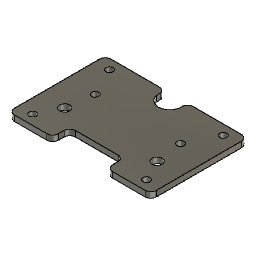
JRCNC0007 v3 (Autodesk Fusion 360 design; units mm, degrees)
Autodesk Fusion 360 part; units mm, degrees
sketch "Sketch1" plane through (0, 0, 0) normal (0, 0, 1) x (1, 0, 0)
  line L0 (-7.8581, 65) -> (-7.8581, 62)
  circle A0 centre (-40, 7) radius 2.5
  line L1 (-32.5, 22) -> (32.5, 22) construction
  line L2 (-40, 61) -> (-40, 7) construction
  arc A1 (19, 8) -> (15, 12) centre (15, 8) ccw
  line L3 (40, 7) -> (40, 61) construction
  arc A2 (-7.8581, 65) -> (-11.7311, 68) centre (-11.7311, 64) ccw
  arc A3 (-50, 4) -> (-46, 0) centre (-46, 4) ccw
  arc A4 (50, 64) -> (46, 68) centre (46, 64) ccw
  line L4 (19, 4) -> (19, 8)
  line L5 (7.8581, 65) -> (7.8581, 62)
  line L6 (-11.7311, 68) -> (-46, 68)
  circle A5 centre (32.5, 22) radius 3.6
  line L7 (-40, 7) -> (40, 7) construction
  line L8 (-30, 41) -> (30, 41) construction
  circle A6 centre (40, 61) radius 2.5
  circle A7 centre (40, 7) radius 2.5
  arc A8 (19, 4) -> (23, 0) centre (23, 4) ccw
  arc A9 (-46, 68) -> (-50, 64) centre (-46, 64) ccw
  line L9 (0, 0) -> (0, 50.832) construction
  arc A10 (11.7311, 68) -> (7.8581, 65) centre (11.7311, 64) ccw
  arc A11 (-15, 12) -> (-19, 8) centre (-15, 8) ccw
  line L10 (-50, 64) -> (-50, 4)
  arc A12 (-7.8581, 62) -> (7.8581, 62) centre (0, 63.5) ccw
  line L11 (15, 12) -> (-15, 12)
  circle A13 centre (-32.5, 22) radius 3.6
  arc A14 (-23, 0) -> (-19, 4) centre (-23, 4) ccw
  line L12 (23, 0) -> (46, 0)
  line L13 (46, 68) -> (11.7311, 68)
  line L14 (-50, 34) -> (50, 34) construction
  circle A15 centre (-30, 41) radius 2.5
  circle A16 centre (-40, 61) radius 2.5
  line L15 (40, 61) -> (-40, 61) construction
  line L16 (50, 4) -> (50, 64)
  arc A17 (46, 0) -> (50, 4) centre (46, 4) ccw
  line L17 (-19, 8) -> (-19, 4)
  line L18 (-46, 0) -> (-23, 0)
  circle A18 centre (30, 41) radius 2.5
  point P0 (-50, 68)
  point P1 (-50, 0)
  point P2 (-50, 0)
  dimension "d1" = 68
  dimension "d3" = 50
  dimension "d4" = 19
  dimension "d5" = 19
  dimension "d6" = 40
  dimension "d7" = 40
  dimension "d8" = 50
  dimension "d9" = 32.5
  dimension "d10" = 32.5
  dimension "d11" = 30
  dimension "d13" = 54
  dimension "d14" = 27
  dimension "d15" = 7
  dimension "d16" = 12
  dimension "d17" = 4
  dimension "d18" = 4
  dimension "d19" = 4
  dimension "d20" = 4
  dimension "d24" = 8
  dimension "d25" = 4.5
  dimension "d27" = 6
  dimension "d28" = 3
  dimension "d29" = 4
  dimension "d30" = 6
  dimension "d32" = 4
  dimension "d35" = 50
  dimension "d36" = 4
  dimension "d37" = 4
  dimension "d38" = 30
  dimension "d39" = 15
  dimension "d40" = 34
  dimension "d44" = 12
  dimension "d45" = 7.2
  dimension "d46" = 5
  dimension "d47" = 30
  dimension "d47" = 30
  constraint horizontal L18
  constraint vertical L16
  constraint horizontal L13
  constraint vertical L10
  constraint coincident P2 P1
  constraint vertical L4
  constraint horizontal L11
  constraint vertical L17
  constraint tangent A8 L18
  constraint horizontal L7
  constraint vertical L3
  constraint horizontal L15
  constraint vertical L2
  constraint coincident L3.end A6.centre
  constraint coincident A0.centre L2.end
  constraint coincident L2.start A16.centre
  constraint coincident L3.start L7.end
  constraint tangent A10 L13
  constraint tangent A14 L18
  constraint tangent A14 L17
  constraint tangent A11 L17
  constraint tangent A11 L11
  constraint tangent A1 L11
  constraint tangent A1 L4
  constraint tangent L4 A8
  constraint coincident A8.end L18
  constraint coincident A1.start L4
  constraint collinear L12 L18
  constraint coincident A2.end L13
  constraint collinear L6 L13
  constraint coincident L1.start A13.centre
  constraint coincident L1.end A5.centre
  constraint parallel L1 L14
  constraint coincident L8.start A15.centre
  constraint coincident L8.end A18.centre
  constraint perpendicular L8 L9
  constraint coincident L14.start L10
  constraint coincident P2 L18
  constraint coincident P2 L10
  constraint tangent A3 L18
  constraint tangent A3 L10
  constraint coincident L14.end L16
  constraint tangent L12 A17
  constraint tangent L16 A17
  constraint tangent A4 L13
  constraint tangent A4 L16
  constraint coincident P0 L6
  constraint coincident P0 L10
  constraint tangent L6 A9
  constraint tangent A9 L10
  constraint perpendicular L5 L15
  constraint perpendicular L0 L15
  constraint equal L0 L5
  constraint tangent A2 L6
  constraint coincident L9.start origin
  constraint coincident L9.start L12
  constraint equal A5 A13
  constraint equal A15 A16
  constraint equal A15 A18
  constraint equal A6 A18
  constraint equal A6 A7
  constraint equal A0 A7
  constraint coincident A1.start L4.end
  measures "d1" distance of P0 P2
  measures "d3" distance of L9 L16
  measures "d4" distance of L4 L9
  measures "d5" distance of L9 L17
  measures "d6" distance of L3 L9
  measures "d7" distance of L2 L9
  measures "d8" distance of L9 L10
  measures "d9" distance of L1.end L9
  measures "d10" distance of L1.start L9
  measures "d11" distance of L8.end L9
  measures "d13" distance of L3.start L3.end
  measures "d14" distance of L3.start L14
  measures "d15" distance of L8 L14
  measures "d16" distance of L1 L14
  measures "d17" radius of A3
  measures "d18" radius of A17
  measures "d19" radius of A4
  measures "d20" radius of A9
  measures "d24" radius of A12
  measures "d25" distance of A12.centre L13
  measures "d27" distance of L0.end L6
  measures "d28" distance of L0.start L6
  measures "d29" radius of A2
  measures "d30" distance of L5.end L13
  measures "d32" radius of A10
  measures "d35" distance of A12.centre L16
  measures "d36" radius of A14
  measures "d37" radius of A8
  measures "d38" distance of A11.start A1.end
  measures "d39" distance of A1.end L9
  measures "d40" distance of L14 L18
  measures "d44" distance of L11 L12
  measures "d45" diameter of A13
  measures "d46" diameter of A15
  measures "d47" distance of L8.start L9
extrude "Extrude1" add sketch "Sketch1" along normal blind 4
equation "d4 = ( 38 / 2 ) * 1 mm"
equation "d9 = ( 65 / 2 ) * 1 mm"
equation "d14 = ( 54 / 2 ) * 1 mm"
